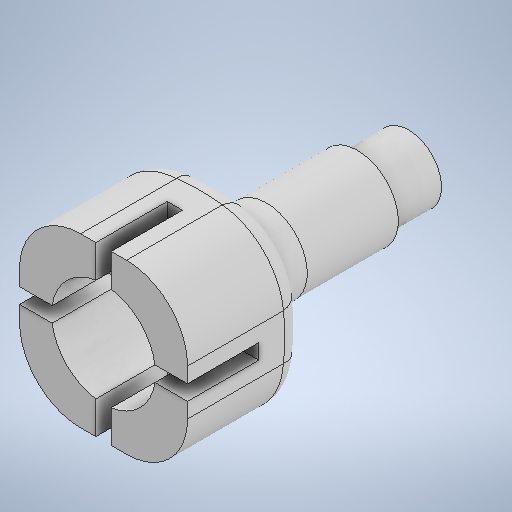
# Autodesk Inventor part: rubik_adapter
Saved by Autodesk Inventor 2025 (Build 290162010, 162A)
## iProperties
Created: 2025-01-16
Part Number: rubik_adapter
Material: Generic
Document SubType Name: Modeling
Designer: aduwa
Density: 1 g/cm^3
Appearance: Default
Author: aduwa
Autodesk Inventor part; units mm, degrees
ref_plane "YZ Plane" through (0, 0, 0) normal (1, 0, 0) x (0, 1, 0)
ref_plane "XZ Plane" through (0, 0, 0) normal (0, 1, 0) x (-1, 0, 0)
ref_plane "XY Plane" through (0, 0, 0) normal (0, 0, 1) x (1, 0, 0)
sketch "Sketch1" plane through (0, 0, 0) normal (0, 0, 1) x (1, 0, 0)
  circle A0 centre (0, 0) radius 5.1
  line L0 (-8.25, 8.25) -> (8.25, 8.25)
  line L1 (8.25, 8.25) -> (8.25, -8.25)
  line L2 (8.25, -8.25) -> (-8.25, -8.25)
  line L3 (-8.25, -8.25) -> (-8.25, 8.25)
  line L4 (-8.25, 8.25) -> (8.25, -8.25) construction
  line L5 (8.25, 8.25) -> (-8.25, -8.25) construction
  line L6 (0.75, -8.25) -> (-0.75, -8.25)
  line L7 (-0.75, -8.25) -> (-0.75, 8.25)
  line L8 (-0.75, 8.25) -> (0.75, 8.25)
  line L9 (0.75, 8.25) -> (0.75, -8.25)
  line L10 (0.75, -8.25) -> (-0.75, 8.25) construction
  line L11 (-0.75, -8.25) -> (0.75, 8.25) construction
  line L12 (8.25, 0.75) -> (-8.25, 0.75)
  line L13 (-8.25, 0.75) -> (-8.25, -0.75)
  line L14 (-8.25, -0.75) -> (8.25, -0.75)
  line L15 (8.25, -0.75) -> (8.25, 0.75)
  line L16 (8.25, 0.75) -> (-8.25, -0.75) construction
  line L17 (-8.25, 0.75) -> (8.25, -0.75) construction
  point P0 (0.75, -5.0446)
  point P1 (5.0446, -0.75)
  point P2 (5.0446, 0.75)
  point P3 (0.75, 5.0446)
  point P4 (-0.75, 5.0446)
  point P5 (-5.0446, 0.75)
  point P6 (-5.0446, -0.75)
  point P7 (-0.75, -5.0446)
  dimension "d0" = 10.2
  dimension "d1" = 16.5
  dimension "d2" = 1.5
  dimension "d3" = 1.5
  dimension "d38" = 16.5
  constraints: 36 end point, 6 midpoint, 6 parallel, 3 horizontal, 3 perpendicular, 2 point on line, 1 centre point, 1 coincident
  measures "d0" diameter of A0
  measures "d1" distance of L1.end L2.end
  measures "d2" distance of L7.end L8.end
  measures "d3" distance of L13.end L12.end
  measures "d38" distance of L0.end L1.end
extrude "Extrusion1" add sketch "Sketch1" against normal blind 11
extrude "Extrusion2" cut sketch "Sketch1" against normal blind 7 contours A0 L14 L9 L12 | A0 L12 L1 L14 | L12 L9 A0 | A0 L9 L14 | L9 L12 L7 A0 | A0 L7 L0 L9 | L9 L14 L7 L12 | L9 L2 L7 A0 | A0 L7 L14 L9 | L7 L12 A0 | L7 L14 A0 L12 | A0 L14 L7 | A0 L14 L3 L12
sketch "Sketch2" plane through (0, 0, -11) normal (0, 0, -1) x (-1, 0, 0)
  circle A0 centre (0, 0) radius 5
  dimension "d8" = 10
  constraints: 1 centre point, 1 coincident
  measures "d8" diameter of A0
extrude "Extrusion3" [suppressed]
fillet "Fillet1" radius 6 4 edges at (8.25, 8.25, -5.5) (8.25, -8.25, -5.5) (-8.25, -8.25, -5.5) (-8.25, 8.25, -5.5)
sketch "Sketch3" plane through (0, 0, -26) normal (0, 0, -1) x (-1, 0, 0)
  line L0 (4, 2.7238) -> (10.2, 2.7238)
  line L1 (10.2, 2.7238) -> (10.2, -2.0551)
  line L2 (10.2, -2.0551) -> (4, -2.0551)
  line L3 (4, -2.0551) -> (4, 2.7238)
  arc A0 (2.5948, 0.1645) -> (2.1, -1.533) centre (0, 0) ccw
  circle A1 centre (0, 0) radius 5 projected
  line L4 (0, 5) -> (10.2, 5)
  line L5 (10.2, 5) -> (10.2, -5)
  line L6 (10.2, -5) -> (0, -5)
  arc A2 (8.25, 2.25) -> (2.25, 8.25) centre (2.25, 2.25) ccw projected
  line L7 (2.25, 8.25) -> (-2.25, 8.25) projected
  arc A3 (-2.25, 8.25) -> (-8.25, 2.25) centre (-2.25, 2.25) ccw projected
  line L8 (-8.25, 2.25) -> (-8.25, -2.25) projected
  arc A4 (-8.25, -2.25) -> (-2.25, -8.25) centre (-2.25, -2.25) ccw projected
  line L9 (-2.25, -8.25) -> (2.25, -8.25) projected
  arc A5 (2.25, -8.25) -> (8.25, -2.25) centre (2.25, -2.25) ccw projected
  line L10 (8.25, -2.25) -> (8.25, 2.25) projected
  line L11 (-2.6, -2.9034) -> (-2.6, 2.8378)
  circle A6 centre (0, 0) radius 2.6
  point P0 (0.75, 5.0446)
  point P1 (2.1, -1.533)
  point P2 (2.5948, 0.1645)
  dimension "d12" = 6.2
  dimension "d13" = 4
  dimension "d14" = 5.2
  constraints: 16 end point, 4 point on circle, 3 tangent, 2 centre point, 2 horizontal, 2 parallel, 1 coincident, 1 concentric, 1 perpendicular, 1 point on line, 1 vertical
  measures "d12" distance of L1.end L2.end
  measures "d13" distance from line of point (0, 0) L3
  measures "d14" diameter of A0
extrude "Extrusion4" [suppressed]
sketch "Sketch4" plane through (-10.2, -5, -26) normal (-1, 0, 0) x (0, 0, 1)
  circle A0 centre (4, 5) radius 1.7
  line L0 (0, 0) -> (0, 10) projected
  point P0 (26, 5)
  point P1 (0, 5)
  point P2 (0, 5)
  dimension "d17" = 3.4
  dimension "d18" = 4
  constraints: 2 horizontal alignment, 2 midpoint, 1 centre point
  measures "d17" diameter of A0
  measures "d18" distance from line of L0 A0.centre
extrude "Extrusion5" [suppressed]
extrude "Extrusion6" [suppressed]
fillet "Fillet2" [suppressed]
fillet "Fillet3" [suppressed]
sketch "Sketch5" plane through (0, 0, -11) normal (0, 0, -1) x (-1, 0, 0)
  arc A0 (8.25, 2.25) -> (2.25, 8.25) centre (2.25, 2.25) ccw projected
  line L0 (2.25, 8.25) -> (-2.25, 8.25) projected
  arc A1 (-2.25, 8.25) -> (-8.25, 2.25) centre (-2.25, 2.25) ccw projected
  line L1 (-8.25, 2.25) -> (-8.25, -2.25) projected
  arc A2 (-8.25, -2.25) -> (-2.25, -8.25) centre (-2.25, -2.25) ccw projected
  line L2 (-2.25, -8.25) -> (2.25, -8.25) projected
  arc A3 (2.25, -8.25) -> (8.25, -2.25) centre (2.25, -2.25) ccw projected
  line L3 (8.25, -2.25) -> (8.25, 2.25) projected
  line L4 (-5.5, 5.5) -> (5.5, 5.5)
  line L5 (5.5, 5.5) -> (5.5, -5.5)
  line L6 (5.5, -5.5) -> (-5.5, -5.5)
  line L7 (-5.5, -5.5) -> (-5.5, 5.5)
  line L8 (-5.5, 5.5) -> (5.5, -5.5) construction
  line L9 (5.5, 5.5) -> (-5.5, -5.5) construction
  point P0 (0, 0)
  dimension "d31" = 11
  dimension "d32" = 11
  constraints: 12 end point, 2 midpoint, 2 parallel, 1 horizontal, 1 perpendicular
  measures "d31" distance of L5.end L6.end
  measures "d32" distance of L4.end L5.end
extrude "Extrusion7" [suppressed]
sketch "Sketch6" plane through (0, 0, -7) normal (0, 0, 1) x (1, 0, 0)
  circle A0 centre (0, 0) radius 5.1
  arc A1 (-2.25, 8.25) -> (-8.25, 2.25) centre (-2.25, 2.25) ccw projected
  line L0 (-2.25, 8.25) -> (2.25, 8.25) projected
  arc A2 (8.25, 2.25) -> (2.25, 8.25) centre (2.25, 2.25) ccw projected
  line L1 (8.25, 2.25) -> (8.25, -2.25) projected
  arc A3 (2.25, -8.25) -> (8.25, -2.25) centre (2.25, -2.25) ccw projected
  line L2 (2.25, -8.25) -> (-2.25, -8.25) projected
  arc A4 (-8.25, -2.25) -> (-2.25, -8.25) centre (-2.25, -2.25) ccw projected
  line L3 (-8.25, -2.25) -> (-8.25, 2.25) projected
  constraints: 1 centre point, 1 coincident
extrude "Extrusion8" cut sketch "Sketch6" against normal blind 2 contours A0
sketch "Sketch12" plane through (0, 0, -11) normal (0, 0, -1) x (-1, 0, 0)
  circle A0 centre (0, 0) radius 8.45
  circle A1 centre (0, 0) radius 9.6
  arc A2 (8.25, 2.25) -> (2.25, 8.25) centre (2.25, 2.25) ccw projected
  line L0 (2.25, 8.25) -> (-2.25, 8.25) projected
  arc A3 (-2.25, 8.25) -> (-8.25, 2.25) centre (-2.25, 2.25) ccw projected
  line L1 (-8.25, 2.25) -> (-8.25, -2.25) projected
  arc A4 (-8.25, -2.25) -> (-2.25, -8.25) centre (-2.25, -2.25) ccw projected
  line L2 (-2.25, -8.25) -> (2.25, -8.25) projected
  arc A5 (2.25, -8.25) -> (8.25, -2.25) centre (2.25, -2.25) ccw projected
  line L3 (8.25, -2.25) -> (8.25, 2.25) projected
  dimension "d54" = 16.9
  dimension "d55" = 19.2
  constraints: 2 centre point, 2 coincident
  measures "d54" diameter of A0
  measures "d55" diameter of A1
extrude "Extrusion14" add sketch "Sketch12" along normal blind 0.001 contours L3 A0 L2 L1 L0 | A0 L0 A2 L3 | L3 A5 L2 A0 | A0 L1 A3 L0 | L2 A4 L1 A0
sketch "Sketch17" plane through (0, 0, -11.001) normal (0, 0, -1) x (-1, 0, 0)
  arc A0 (-1.833, 2.05) -> (1.833, 2.05) centre (0, 0) ccw
  line L0 (-2.2253, -2.75) -> (2.0609, -2.75)
  circle A1 centre (0, 0) radius 4
  line L1 (-1.833, 2.05) -> (1.833, 2.05)
  dimension "d74" = 5.5
  dimension "d75" = 8
  dimension "d76" = 4.8
  constraints: 4 end point, 2 centre point, 2 coincident, 2 point on circle, 1 tangent
  measures "d74" diameter of A0
  measures "d75" diameter of A1
  measures "d76" distance between parallel lines of L1 L0
extrude "Extrusion19" add sketch "Sketch17" along normal blind 18.94
sketch "Sketch18" plane through (0, 0, -29.941) normal (0, 0, -1) x (-1, 0, 0)
  circle A0 centre (0, 0) radius 3.25
  circle A1 centre (0, 0) radius 4
  dimension "d79" = 6.5
  constraints: 2 centre point, 1 coincident
  measures "d79" diameter of A0
extrude "Extrusion20" cut sketch "Sketch18" against normal blind 5
fillet "Fillet5" radius 5 1 edges at (4, 0, -11.001)
fillet "Fillet6" radius 2 22 edges at (6.4926, 6.4926, -11.001) (8.1499, 3.3415, -11.0047) (3.3415, 8.1499, -11.0047) (3.342, 8.1498, -11.001) (8.1498, 3.342, -11.001) (0, 8.25, -11.0576) (-8.1499, 3.3415, -11.0047) (-3.3415, 8.1499, -11.0047) (-6.4926, 6.4926, -11.001) (-8.25, -2.2498, -11.0212) (-8.25, -1.125, -11.0466) (-8.25, 1.1252, -11.0466) (-3.3415, -8.1499, -11.0047) (-8.1499, -3.3415, -11.0047) (-6.4926, -6.4926, -11.001) (0, -8.25, -11.0576) (3.3415, -8.1499, -11.0047) (8.1499, -3.3415, -11.0047) (3.342, -8.1498, -11.001) (8.1498, -3.342, -11.001) (6.4926, -6.4926, -11.001) (8.25, 0, -11.0576)
sketch "Sketch19" plane through (0, 0, -29.941) normal (0, 0, -1) x (-1, 0, 0)
  line L0 (-0.5, -1.7023) -> (0.5, -1.7023)
  line L1 (0.5, -1.7023) -> (0.5, -4.2576)
  line L2 (0.5, -4.2576) -> (-0.5, -4.2576)
  line L3 (-0.5, -4.2576) -> (-0.5, -1.7023)
  line L4 (-0.5, -1.7023) -> (0.5, -4.2576) construction
  line L5 (0.5, -1.7023) -> (-0.5, -4.2576) construction
  point P0 (0, 0)
  point P1 (0, -2.9799)
  point P2 (0, -2.9799)
  dimension "d84" = 1
  constraints: 12 end point, 3 midpoint, 2 parallel, 1 horizontal, 1 perpendicular, 1 other
  measures "d84" distance of L2.end L1.end
extrude "Extrusion21" cut sketch "Sketch19" against normal blind 3
body "Solid1"
